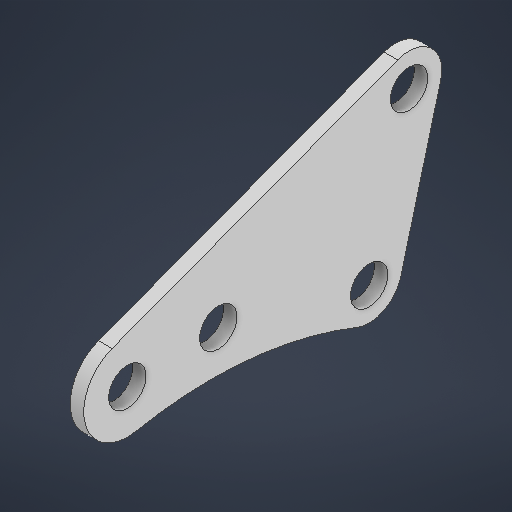
# Autodesk Inventor part: rotationmount
Saved by Autodesk Inventor 2025.2 (Build 292293000, 293)
## iProperties
Created: 2025-04-17
Part Number: rotationmount
Material: Generic
Document SubType Name: Modeling
Designer: roejo
Density: 1 g/cm^3
Appearance: Default
Author: roejo
Autodesk Inventor part; units mm, degrees
ref_plane "YZ Plane" through (0, 0, 0) normal (1, 0, 0) x (0, 1, 0)
ref_plane "XZ Plane" through (0, 0, 0) normal (0, 1, 0) x (-1, 0, 0)
ref_plane "XY Plane" through (0, 0, 0) normal (0, 0, 1) x (1, 0, 0)
sketch "Sketch1" plane through (0, 0, 0) normal (1, 0, 0) x (0, 1, 0)
  circle A0 centre (0, 0) radius 2.1844
  circle A1 centre (0, 0) radius 3.81
  circle A2 centre (3.8397, 28.1547) radius 2.1844
  circle A3 centre (3.8397, 28.1547) radius 5.08
  line L0 (0, 0) -> (16.51, 0) construction
  circle A4 centre (17.5016, -4.6538) radius 2.1844
  line L1 (0, 0) -> (16.51, 0) construction
  circle A5 centre (4.5215, 17.5685) radius 2.1844
  circle A6 centre (4.5215, 17.5685) radius 3.81
  circle A7 centre (17.5016, -4.6538) radius 3.81
  line L2 (0, 0) -> (12.7, 0) construction
  line L3 (-0.9791, -3.6821) -> (16.5226, -8.3359)
  line L4 (8.5961, 29.9387) -> (21.069, -3.3158)
  arc A8 (-3.5374, 1.4152) -> (-1.1438, 27.1693) centre (-45.8278, 18.334) ccw
  point P0 (-1.2195, 28.6143)
  point P1 (-3.7944, 0.3447)
  dimension "d0" = 4.3688
  dimension "d1" = 7.62
  dimension "d3" = 4.3688
  dimension "d4" = 10.16
  dimension "d8" = 4.3688
  dimension "d11" = 4.3688
  dimension "d12" = 7.62
  dimension "d13" = 7.62
  constraints: 10 end point, 10 point on circle, 9 centre point, 6 tangent, 5 coincident, 3 horizontal
  measures "d0" diameter of A0
  measures "d1" diameter of A1
  measures "d3" diameter of A2
  measures "d4" diameter of A3
  measures "d8" diameter of A4
  measures "d11" diameter of A5
  measures "d12" diameter of A6
  measures "d13" diameter of A7
extrude "Extrusion1" add sketch "Sketch1" along normal blind 1.5875 contours A1 | A1 A8 A3 L4 A7 L3 | A3 | A7 | A6
body "Solid1"
